# Autodesk Inventor part: standoff_20mm
Saved by Autodesk Inventor 2021 (Build 250183000, 183)
## iProperties
Created: 2021-01-16
Part Number: standoff_20mm
Material: Stainless Steel
Document SubType Name: Modeling
Designer: User
Density: 8 g/cm^3
Appearance: Semi-Polished
Author: User
Autodesk Inventor part; units mm, degrees
ref_plane "YZ Plane" through (0, 0, 0) normal (1, 0, 0) x (0, 1, 0)
ref_plane "XZ Plane" through (0, 0, 0) normal (0, 1, 0) x (-1, 0, 0)
ref_plane "XY Plane" through (0, 0, 0) normal (0, 0, 1) x (1, 0, 0)
sketch "Sketch1" plane through (0, 0, 0) normal (0, 1, 0) x (-1, 0, 0)
  line L0 (0, -3.0022) -> (-2.6, -1.5011)
  line L1 (-2.6, -1.5011) -> (-2.6, 1.5011)
  line L2 (-2.6, 1.5011) -> (0, 3.0022)
  line L3 (0, 3.0022) -> (2.6, 1.5011)
  line L4 (2.6, 1.5011) -> (2.6, -1.5011)
  line L5 (2.6, -1.5011) -> (0, -3.0022)
  circle A0 centre (0, 0) radius 1
  dimension "d0" = 5.2
  dimension "d1" = 2
  constraints: 12 end point, 2 coincident, 1 centre point, 1 vertical alignment, 13 other
  measures "d0" distance between parallel lines of L0 L3
  measures "d1" diameter of A0
extrude "Extrusion1" add sketch "Sketch1" along normal blind 6
body "Solid1"
